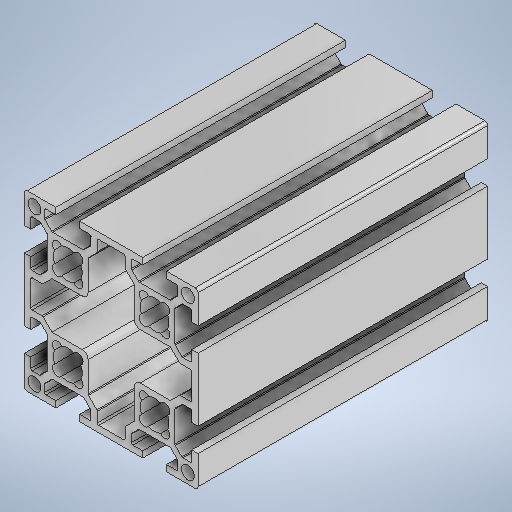
# Autodesk Inventor part: Perfil 60×60 8 rasgos_001
Saved by Autodesk Inventor 2026 (Build 300175000, 175)
## iProperties
Created: 2025-04-07
Part Number: Perfil 60×60 8 rasgos_001
Material: Aluminum 6061
Document SubType Name: Modeling
Designer: Carlos Dias
Density: 2.7 g/cm^3
Appearance: Aluminum - Polished
Author: Carlos Dias
Autodesk Inventor part; units mm, degrees
ref_plane "YZ Plane" through (0, 0, 0) normal (1, 0, 0) x (0, 1, 0)
ref_plane "XZ Plane" through (0, 0, 0) normal (0, 1, 0) x (-1, 0, 0)
ref_plane "XY Plane" through (0, 0, 0) normal (0, 0, 1) x (1, 0, 0)
sketch "Sketch1" plane through (0, 0, 0) normal (0, 0, 1) x (1, 0, 0)
  circle A0 centre (-15, 15) radius 5 construction
  circle A1 centre (-26.5, 26.5) radius 2.25
  line L0 (-30, 30) -> (0, 0) construction
  circle A2 centre (-18.5355, 18.5355) radius 1.75 construction
  line L1 (-22, 22) -> (-22, 8) construction
  line L2 (-22, 22) -> (-8, 22) construction
  line L3 (-30, 0) -> (0, 30) construction
  line L4 (-8, 22) -> (-8, 8) construction
  line L5 (-22, 8) -> (-8, 8) construction
  line L6 (-30, 30) -> (-30, 19.1)
  line L7 (-24.5556, 23) -> (-22, 20.4444)
  line L8 (-30, 19.1) -> (-27.8, 19.1)
  line L9 (-27.8, 23) -> (-27.8, 19.1)
  line L10 (-27.8, 23) -> (-24.5556, 23)
  line L11 (-23, 24.5556) -> (-20.4444, 22)
  line L12 (-23, 27.8) -> (-23, 24.5556)
  line L13 (-30, 30) -> (-19.1, 30)
  line L14 (-19.1, 27.8) -> (-19.1, 30)
  line L15 (-19.1, 27.8) -> (-23, 27.8)
  arc A3 (-17.1006, 19.5373) -> (-19.5373, 17.1006) centre (-18.5355, 18.5355) ccw
  arc A4 (-19.5373, 17.1006) -> (-20, 15) centre (-15, 15) ccw
  arc A5 (-15, 20) -> (-17.1006, 19.5373) centre (-15, 15) ccw
  arc A6 (-20, 15) -> (-19.5373, 12.8994) centre (-15, 15) ccw
  arc A7 (-19.5373, 12.8994) -> (-17.1006, 10.4627) centre (-18.5355, 11.4645) ccw
  arc A8 (-17.1006, 10.4627) -> (-15, 10) centre (-15, 15) ccw
  arc A9 (-15, 10) -> (-12.8994, 10.4627) centre (-15, 15) ccw
  arc A10 (-12.8994, 10.4627) -> (-10.4627, 12.8994) centre (-11.4645, 11.4645) ccw
  arc A11 (-10.4627, 12.8994) -> (-10, 15) centre (-15, 15) ccw
  arc A12 (-10, 15) -> (-10.4627, 17.1006) centre (-15, 15) ccw
  arc A13 (-10.4627, 17.1006) -> (-12.8994, 19.5373) centre (-11.4645, 18.5355) ccw
  arc A14 (-12.8994, 19.5373) -> (-15, 20) centre (-15, 15) ccw
  line L16 (-22, 9.5556) -> (-24.5556, 7)
  line L17 (-27.8, 7) -> (-24.5556, 7)
  line L18 (-27.8, 10.9) -> (-27.8, 7)
  line L19 (-30, 10.9) -> (-27.8, 10.9)
  line L20 (-30, 10.9) -> (-30, 0)
  line L21 (-22, 20.4444) -> (-22, 9.5556)
  line L22 (-20.4444, 8) -> (-23.6444, 4.8)
  line L23 (-27.8, 4.8) -> (-23.6444, 4.8)
  line L24 (-27.8, 4.8) -> (-27.8, 0)
  line L25 (-27.8, 0) -> (-30, 0)
  line L26 (-7, 24.5556) -> (-9.5556, 22)
  line L27 (-20.4444, 8) -> (-8, 8)
  line L28 (-8, 20.4444) -> (-4.8, 23.6444)
  line L29 (-8, 20.4444) -> (-8, 8)
  line L30 (-9.5556, 22) -> (-20.4444, 22)
  line L31 (-7, 24.5556) -> (-7, 27.8)
  line L32 (-4.8, 23.6444) -> (-4.8, 27.8)
  line L33 (-10.9, 27.8) -> (-7, 27.8)
  line L34 (-10.9, 30) -> (-10.9, 27.8)
  line L35 (-10.9, 30) -> (0, 30)
  line L36 (-4.8, 27.8) -> (0, 27.8)
  line L37 (0, 27.8) -> (0, 30)
  point P0 (-15, 15)
  point P1 (-15, 20)
  point P2 (-10, 15)
  point P3 (-15, 10)
  dimension "d0" = 10
  dimension "d1" = 15
  dimension "d2" = 15
  dimension "d3" = 4.5
  dimension "d4" = 26.5
  dimension "d5" = 26.5
  dimension "d6" = 30
  dimension "d7" = 30
  dimension "d8" = 3.5
  dimension "d9" = 8
  dimension "d10" = 4.1
  dimension "d11" = 1.1
  dimension "d12" = 2.2
  dimension "d13" = 1.25
  dimension "d14" = 4.1
  dimension "d17" = 360
  dimension "d19" = 1.1
  dimension "d20" = 2.2
  dimension "d21" = 1.1
  constraints: 76 end point, 31 point on circle, 15 centre point, 14 equal length, 12 vertical, 11 horizontal, 11 point on line, 4 vertical alignment, 3 collinear, 3 concentric, 3 horizontal alignment, 3 parallel, 2 midpoint, 1 coincident, 1 perpendicular, 44 other
  measures "d0" diameter of A0
  measures "d1" horizontal distance of point (0, 0) A0.centre
  measures "d2" horizontal distance of point (0, 0) A0.centre
  measures "d3" diameter of A1
  measures "d4" horizontal distance of point (0, 0) A1.centre
  measures "d5" horizontal distance of point (0, 0) A1.centre
  measures "d6" horizontal distance of point (0, 0) L0.start
  measures "d7" horizontal distance of point (0, 0) L0.start
  measures "d8" diameter of A2
  measures "d9" distance from line of L0.start L1
  measures "d10" vertical distance of point (-15, 15) L6.end
  measures "d11" distance between parallel lines of L0 L7
  measures "d12" distance of L6.end L8.end
  measures "d13" distance edge to line of A1 L10
  measures "d14" horizontal distance of point (-15, 15) L13.end
  measures "d19" distance between parallel lines of L3 L16
  measures "d20" distance between parallel lines of L17 L23
  measures "d21" distance between parallel lines of L3 L26
extrude "Extrusion1" add sketch "Sketch1" along normal mid plane 100
fillet "Fillet1" radius 1 1 edges at (-30, 30, 0)
fillet "Fillet2" radius 0.5 17 edges at (-9.5556, 22, 0) (-7, 24.5556, 0) (-22, 9.5556, 0) (-24.5556, 7, 0) (-27.8, 7, 0) (-20.4444, 22, 0) (-23, 24.5556, 0) (-7, 27.8, 0) (-24.5556, 23, 0) (-22, 20.4444, 0) (-23, 27.8, 0) (-27.8, 23, 0) (-4.8, 23.6444, 0) (-8, 20.4444, 0) (-4.8, 27.8, 0) (-23.6444, 4.8, 0) (-27.8, 4.8, 0)
fillet "Fillet3" radius 2 1 edges at (-8, 8, 0)
mirror "Mirror1" about plane through (0, 0, 0) normal (1, 0, 0) of "Extrusion1", "Fillet1", "Fillet2", "Fillet3"
mirror "Mirror2" about plane through (0, 0, 0) normal (0, 1, 0) of "Extrusion1", "Fillet1", "Fillet2", "Fillet3", "Mirror1"
equation "\"d2\" = d1"
equation "\"d5\" = d4"
equation "\"d7\" = d6"
equation "\"d11\" = 0.5 * d12"
equation "\"d14\" = d10"
equation "\"d19\" = 0.5 * d12"
equation "\"d20\" = d12"
equation "\"d21\" = 0.5 * d12"
body "Solid1"
